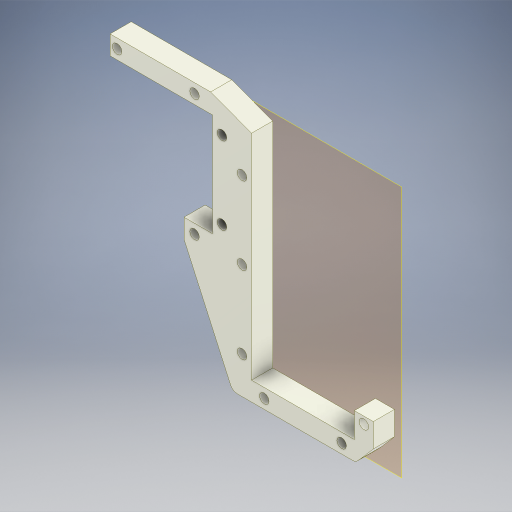
# Autodesk Inventor part: leg_ver2
Saved by Autodesk Inventor 2024 (Build 280153000, 153)
## iProperties
Created: 2024-09-04
Part Number: leg_ver2
Material: PMMA 플라스틱
Document SubType Name: Modeling
Designer: msi
Density: 1.188 g/cm^3
Appearance: 매끄러움 - 아이보리색
Author: msi
Autodesk Inventor part; units mm, degrees
ref_plane "YZ Plane" through (0, 0, 0) normal (1, 0, 0) x (0, 1, 0)
ref_plane "XZ Plane" through (0, 0, 0) normal (0, 1, 0) x (-1, 0, 0)
ref_plane "XY Plane" through (0, 0, 0) normal (0, 0, 1) x (1, 0, 0)
ref_plane "작업 평면1" through (0, 0, 0) normal (0, 0, 1) x (1, 0, 0)
sketch "스케치1" plane through (0, 0, 0) normal (0, 0, 1) x (1, 0, 0)
  line L0 (-85.3, -15) -> (-85.3, -11.5) projected
  line L1 (-85.3, -15) -> (-79.3, -20.1) projected
  line L2 (-79.3, -20.1) -> (-26.2, -20.1) projected
  line L3 (-26.2, -20.1) -> (-20.2, -15) projected
  line L4 (-20.2, -15) -> (-20.2, 15) projected
  line L5 (-20.2, 15) -> (-26.2, 20.1) projected
  line L6 (-26.2, 20.1) -> (-79.3, 20.1) projected
  line L7 (-79.3, 20.1) -> (-85.3, 15) projected
  line L8 (-85.3, 11.5) -> (-85.3, 15) projected
  arc A0 (-82.3, 14.5) -> (-85.3, 11.5) centre (-82.3, 11.5) ccw projected
  line L9 (-28.8, 14.5) -> (-82.3, 14.5) projected
  arc A1 (-25.8, 11.5) -> (-28.8, 14.5) centre (-28.8, 11.5) ccw projected
  line L10 (-25.8, -11.5) -> (-25.8, 11.5) projected
  arc A2 (-28.8, -14.5) -> (-25.8, -11.5) centre (-28.8, -11.5) ccw projected
  line L11 (-82.3, -14.5) -> (-28.8, -14.5) projected
  arc A3 (-85.3, -11.5) -> (-82.3, -14.5) centre (-82.3, -11.5) ccw projected
  circle A4 centre (-74.8, 17.3) radius 1.35 projected
  circle A5 centre (-52.8, 17.3) radius 1.35 projected
  circle A6 centre (-30.8, 17.3) radius 1.35 projected
  circle A7 centre (-23, 11) radius 1.35 projected
  circle A8 centre (-74.8, -17.3) radius 1.35 projected
  circle A9 centre (-52.8, -17.3) radius 1.35 projected
  circle A10 centre (-30.8, -17.3) radius 1.35 projected
  circle A11 centre (-23, -11) radius 1.35 projected
  line L12 (-15, 14.5) -> (-11.5, 14.5) projected
  line L13 (-15, 14.5) -> (-20.1, 8.5) projected
  line L14 (-20.1, 8.5) -> (-20.1, -44.6) projected
  line L15 (-20.1, -44.6) -> (-15, -50.6) projected
  line L16 (-15, -50.6) -> (15, -50.6) projected
  line L17 (15, -50.6) -> (20.1, -44.6) projected
  line L18 (20.1, -44.6) -> (20.1, 8.5) projected
  line L19 (20.1, 8.5) -> (15, 14.5) projected
  line L20 (11.5, 14.5) -> (15, 14.5) projected
  arc A12 (14.5, 11.5) -> (11.5, 14.5) centre (11.5, 11.5) ccw projected
  line L21 (14.5, -42) -> (14.5, 11.5) projected
  arc A13 (11.5, -45) -> (14.5, -42) centre (11.5, -42) ccw projected
  line L22 (-11.5, -45) -> (11.5, -45) projected
  arc A14 (-14.5, -42) -> (-11.5, -45) centre (-11.5, -42) ccw projected
  line L23 (-14.5, 11.5) -> (-14.5, -42) projected
  arc A15 (-11.5, 14.5) -> (-14.5, 11.5) centre (-11.5, 11.5) ccw projected
  circle A16 centre (17.3, 4) radius 1.35 projected
  circle A17 centre (17.3, -18) radius 1.35 projected
  circle A18 centre (17.3, -40) radius 1.35 projected
  circle A19 centre (11, -47.8) radius 1.35 projected
  circle A20 centre (-17.3, 4) radius 1.35 projected
  circle A21 centre (-17.3, -18) radius 1.35 projected
  circle A22 centre (-17.3, -40) radius 1.35 projected
  circle A23 centre (-11, -47.8) radius 1.35 projected
  arc A24 (-14.6, -42) -> (-11.5, -45.1) centre (-11.5, -42) ccw
  line L24 (-11.5, -45.1) -> (11.5, -45.1)
  arc A25 (11.5, -45.1) -> (14.6, -42) centre (11.5, -42) ccw
  line L25 (14.6, -42) -> (14.6, 11.5)
  arc A26 (14.6, 11.5) -> (12.5954, 14.4) centre (11.5, 11.5) ccw
  line L26 (12.5954, 14.4) -> (14.9538, 14.4)
  line L27 (14.9538, 14.4) -> (20, 8.4632)
  line L28 (20, 8.4632) -> (20, -44.5632)
  line L29 (14.9538, -50.5) -> (-14.9538, -50.5)
  line L30 (-14.6, 11.5) -> (-14.6, -42)
  arc A27 (-25.7, 11.5) -> (-28.8, 14.6) centre (-28.8, 11.5) ccw
  line L31 (-28.8, 14.6) -> (-82.3, 14.6)
  arc A28 (-82.3, 14.6) -> (-85.2, 12.5954) centre (-82.3, 11.5) ccw
  line L32 (-85.2, 12.5954) -> (-85.2, 14.9538)
  line L33 (-85.2, 14.9538) -> (-79.2632, 20)
  line L34 (-79.2632, 20) -> (-26.2368, 20)
  line L35 (-20.3, -14.9538) -> (-26.2368, -20)
  line L36 (-26.2368, -20) -> (-79.2632, -20)
  line L37 (-79.2632, -20) -> (-85.2, -14.9538)
  line L38 (-85.2, -14.9538) -> (-85.2, -12.5954)
  arc A29 (-85.2, -12.5954) -> (-82.3, -14.6) centre (-82.3, -11.5) ccw
  line L39 (-82.3, -14.6) -> (-28.8, -14.6)
  arc A30 (-28.8, -14.6) -> (-25.7, -11.5) centre (-28.8, -11.5) ccw
  line L40 (-25.7, -11.5) -> (-25.7, 11.5)
  line L41 (-14.6, 15.6629) -> (-14.6, -30)
  circle A31 centre (-23, -11) radius 1.35
  circle A32 centre (-23, 11) radius 1.35
  circle A33 centre (-17.3, -18) radius 1.35
  circle A34 centre (-17.3, 4) radius 1.35
  line L42 (-28.8, 14.6) -> (-54.8, 14.6)
  line L43 (-54.8, 14.6) -> (-54.8, 20)
  line L44 (-54.8, 20) -> (-28.8, 20)
  line L45 (-28.8, 20) -> (-28.8, 14.6)
  line L46 (-28.8, 14.6) -> (-25.7, 14.6)
  line L47 (-28.8, 19.6629) -> (-28.8, 14.6)
  line L48 (-28.8, -14.6) -> (-33.8, -14.6)
  line L49 (-33.8, -14.6) -> (-33.8, -20)
  line L50 (-33.8, -20) -> (-28.8, -20)
  line L51 (-28.8, -20) -> (-28.8, -14.6)
  line L52 (-28.8, -14.6) -> (-25.659, -14.6)
  line L53 (-26.2368, -20) -> (-28.8, -20)
  line L54 (-28.8, -20) -> (-28.8, -14.6)
  line L55 (-14.6, -30) -> (-14.6, -45.1)
  line L56 (-14.6, -50.5) -> (-20, -50.5)
  line L57 (-14.5, -50.5) -> (-7.5, -50.5)
  line L58 (-7.5, -50.5) -> (-7.5, -45.1)
  line L59 (-7.5, -45.1) -> (-14.5, -45.1)
  line L60 (-14.5, -45.1) -> (-14.5, -50.5)
  line L61 (-20, -50.5) -> (-33.8, -20)
  line L62 (-25.659, -14.6) -> (-25.659, 14.6)
  line L63 (-14.5, -45.1) -> (-14.6, -45.1)
  line L64 (-7.5, -45.1) -> (14.9538, -45.1)
  line L65 (14.9538, -45.1) -> (14.9538, -50.5)
  line L66 (14.9538, -50.5) -> (-7.5, -50.5)
  line L67 (-7.5, -50.5) -> (-7.5, -45.1)
  circle A35 centre (11, -47.8) radius 1.35
  line L68 (14.6, -42) -> (20, -42)
  line L69 (20, -42) -> (20, -45.1)
  line L70 (20, -45.1) -> (14.6, -45.1)
  line L71 (14.6, -45.1) -> (14.6, -42)
  line L72 (20, -42) -> (14.6, -42)
  line L73 (14.6, -42) -> (14.6, -38)
  line L74 (14.6, -38) -> (20, -38)
  line L75 (20, -38) -> (20, -42)
  line L76 (20, -45.1) -> (14.9538, -50.5)
  circle A36 centre (-30.8, -17.3) radius 1.35
  circle A37 centre (-17.3, -40) radius 1.35
  circle A38 centre (-11, -47.8) radius 1.35
  circle A39 centre (17.3, -40) radius 1.35
  line L77 (-25.7, 14.6) -> (-25.659, 14.6)
  line L78 (-26.2368, 20) -> (-14.6, 15.6629)
  point P0 (0, 0)
  point P1 (-14.6, -30)
  point P2 (-28.8, 14.6)
  point P3 (-28.8, -14.6)
  point P4 (-26.2368, -20)
  point P5 (-26.0824, -20)
  point P6 (-33.7548, -20.1)
  point P7 (16.4054, -48.9466)
  point P8 (20, -44.7176)
  point P9 (-11.5, -45.1)
  point P10 (-14.6, -30)
  dimension "d0" = 0.1
  dimension "d1" = 0.1
  dimension "d3" = 2.7
  dimension "d4" = 2.7
  dimension "d5" = 2.7
  dimension "d6" = 2.7
  dimension "d9" = 26
  dimension "d10" = 5
  dimension "d11" = 7
  dimension "d16" = 4
  constraints: 110 end point, 16 centre point, 16 point on circle, 14 parallel, 9 coincident, 8 horizontal, 8 perpendicular, 8 point on line, 5 concentric, 19 other
  measures "d0" distance between parallel lines of L23 L30
  measures "d1" distance between parallel lines of L10 L40
  measures "d3" diameter of A31
  measures "d4" diameter of A32
  measures "d5" diameter of A33
  measures "d6" diameter of A34
  measures "d9" distance of L43.end L44.end
  measures "d10" distance of L50.end L49.end
  measures "d11" distance of L59.end L58.end
  measures "d16" distance of L72.end L73.end
extrude "돌출4" add sketch "스케치1" along normal blind 6 contours L61 L36 L51 L52 L62 L77 L46 L45 L34 L78 L5 L4 L3 L2 | L2 L3 L4 L5 L78 L41 L12 L13 L14 L15 L56 L61 | L49 L39 L51 L36 | L15 L14 L13 L12 L41 L30 L55 L63 L60 L29 L56 | L76 L65 L70 L17 | L60 L59 L24 L58 L29 | L45 L31 L43 L34 | L70 L64 L71 L68 L28 L69 L17 | L29 L58 L24 L64 L65 | L68 L25 L74 L28
fillet "모깎기3" radius 2 2 edges at (-20, -50.5, 3) (14.9538, -50.5, 3)
